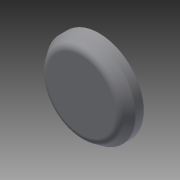
# Autodesk Inventor part: coating
Saved by Autodesk Inventor 2015 SP1 (Build 190203100, 203)
## iProperties
Created: 2015-02-17
Part Number: coating
Material: Generic
Document SubType Name: Modeling
Designer: Jostein
Density: 1 g/cm^3
Appearance: Default
Author: Jostein
Autodesk Inventor part; units mm, degrees
ref_plane "YZ Plane" through (0, 0, 0) normal (1, 0, 0) x (0, 1, 0)
ref_plane "XZ Plane" through (0, 0, 0) normal (0, 1, 0) x (-1, 0, 0)
ref_plane "XY Plane" through (0, 0, 0) normal (0, 0, 1) x (1, 0, 0)
sketch "Sketch1" plane through (0, 0, 0) normal (0, 0, 1) x (1, 0, 0)
  line L0 (320, 126) -> (320, 70)
  line L1 (320, 70) -> (285.9746, 21.3454)
  arc A0 (245, 0) -> (285.9746, 21.3454) centre (245, 50) ccw
  line L2 (245, 0) -> (0, 0)
  line L3 (320, 129) -> (320, 126)
  line L4 (0, -2) -> (245, -2)
  arc A1 (245, -2) -> (287.6135, 20.1992) centre (245, 50) ccw
  line L5 (287.6135, 20.1992) -> (322, 69.3701)
  line L6 (322, 69.3701) -> (322, 126)
  line L7 (322, 126) -> (322, 129)
  line L8 (322, 129) -> (320, 129)
  line L9 (0, -25.8) -> (0, 154.8) construction
  line L10 (0, 0) -> (0, -2)
  point P0 (0, 0)
  dimension "d0" = 2
  dimension "d1" = 30.4542
  constraints: 22 end point, 4 point on circle, 3 vertical, 2 centre point, 2 horizontal, 2 point on line, 1 collinear, 1 parallel, 1 tangent, 13 other
  measures "d0" distance between parallel lines of L1 L5
  measures "d1" distance from line of L6.end L1
revolve "Revolution1" add sketch "Sketch1" angle 360 about axis through (0, -25.8, 0) along (0, 1, 0)
sketch "Sketch2" plane through (0, 0, 0) normal (0, 1, 0) x (1, 0, 0)
  circle A0 centre (0, -138) radius 12 projected
  circle A1 centre (119.5115, 69) radius 12 projected
  circle A2 centre (-119.5115, 69) radius 12 projected
  point P0 (0, 0)
extrude "Extrusion1" cut sketch "Sketch2" against normal through all
body "Solid1"
